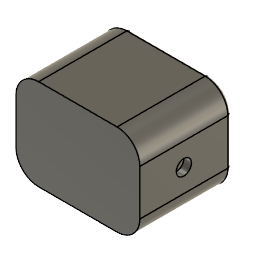
gimbal (Autodesk Fusion 360 archive; units mm, degrees)
design "camera"
Autodesk Fusion 360 part; units mm, degrees
sketch "Sketch1" plane through (0, 0, 0) normal (0, 0, 1) x (1, 0, 0)
  line L0 (20.4, -15) -> (-20.4, -15)
  line L1 (-20.4, -15) -> (-20.4, 15)
  line L2 (-20.4, 15) -> (20.4, 15)
  line L3 (20.4, 15) -> (20.4, -15)
  line L4 (20.4, -15) -> (-20.4, 15) construction
  line L5 (-20.4, -15) -> (20.4, 15) construction
  dimension "d1" = 30
  dimension "d2" = 40.8
  constraint horizontal L0
  constraint perpendicular L0 L1
  constraint parallel L0 L2
  constraint parallel L1 L3
  constraint coincident L4 origin
  constraint coincident L5 origin
  measures "d1" distance of L0.end L1.end
  measures "d2" distance of L1.end L2.end
extrude "Extrude1" add sketch "Sketch1" along normal blind 30 makes body 1
fillet "Fillet4" radius 7.5 4 edges at (20.4, 0, 30) (-20.4, 0, 30) (20.4, 0, 0) (-20.4, 0, 0) on bodies 1
hole "Hole1" at (0, 15, 15) direction (0, -1, 0) diameter 20 depth 15 tip angle 118 bodies 1
ref_plane "WorkPlane1" through (0, 20, 0) normal (0, 1, 0) x (0, 0, 1)
sketch "Sketch4" plane through (0, 15, 0) normal (0, 1, 0) x (-1, 0, 0)
  circle A0 centre (0, 15) radius 10
  arc A1 (12.9, 0) -> (20.4, 7.5) centre (12.9, 7.5) ccw
  line L0 (20.4, 7.5) -> (20.4, 22.5)
  arc A2 (20.4, 22.5) -> (12.9, 30) centre (12.9, 22.5) ccw
  line L1 (12.9, 30) -> (-12.9, 30)
  arc A3 (-12.9, 30) -> (-20.4, 22.5) centre (-12.9, 22.5) ccw
  line L2 (-20.4, 22.5) -> (-20.4, 7.5)
  arc A4 (-20.4, 7.5) -> (-12.9, 0) centre (-12.9, 7.5) ccw
  line L3 (-12.9, 0) -> (12.9, 0)
  circle A5 centre (0, 15) radius 10
  constraint concentric A0 A5
extrude "Extrude4" add sketch "Sketch4" along normal blind 1 separate body contours A0 A5 makes body 2
ref_plane "WorkPlane3" through (0, 16, 15) normal (0, 1, 0) x (-1, 0, 0)
sketch "Sketch5" plane through (0, 16, 0) normal (0, 1, 0) x (1, 0, 0)
  circle A0 centre (0, -15) radius 8.2462
extrude "Extrude5" add sketch "Sketch5" along normal blind 2 bodies 2
fillet "Fillet5" radius 0.9 1 edges at (-7.6882, 18, 17.982) on bodies 2
fillet "Fillet6" radius 0.4 1 edges at (9.3233, 16, 11.3838) on bodies 2
fillet "Fillet7" radius 1 1 faces at (-16.924, 15, 14.7509) on bodies 1
ref_plane "WorkPlane4" through (0, 15, 15) normal (0, 1, 0) x (-1, 0, 0)
sketch "Sketch6" plane through (0, 15, 0) normal (0, 1, 0) x (1, 0, 0)
  circle A0 centre (-13, -25) radius 2
  dimension "d42" = 4
  measures "d42" diameter of A0
extrude "Extrude6" cut sketch "Sketch6" against normal blind 0.5 bodies 1
hole "Hole2" at (20.4, -0.5, 15) direction (-1, 0, 0) diameter 5 depth 2.5 tip angle 180 bodies 1
hole "Hole3" at (-20.4, -0.5, 15) direction (1, 0, 0) diameter 5 depth 2.5 tip angle 180 bodies 1

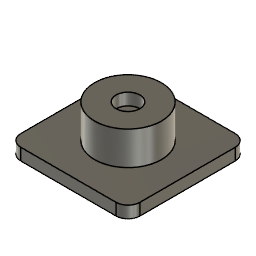
design "gimble stand"
Autodesk Fusion 360 part; units mm, degrees
sketch "Sketch1" plane through (0, 0, 0) normal (0, 0, 1) x (1, 0, 0)
  line L0 (25, -25) -> (-25, -25)
  line L1 (-25, -25) -> (-25, 25)
  line L2 (-25, 25) -> (25, 25)
  line L3 (25, 25) -> (25, -25)
  line L4 (25, -25) -> (-25, 25) construction
  line L5 (-25, -25) -> (25, 25) construction
  dimension "d1" = 50
  dimension "d2" = 50
  constraint horizontal L0
  constraint perpendicular L0 L1
  constraint parallel L0 L2
  constraint parallel L1 L3
  constraint coincident L4 origin
  constraint coincident L5 origin
  measures "d1" distance of L1.end L2.end
  measures "d2" distance of L0.end L1.end
extrude "Extrude1" add sketch "Sketch1" along normal blind 5
ref_plane "WorkPlane1" through (0, 0, 5) normal (0, 0, 1) x (1, 0, 0)
sketch "Sketch2" plane through (0, 0, 5) normal (0, 0, 1) x (1, 0, 0)
  circle A0 centre (0, 0) radius 14
  dimension "d6" = 28
  constraint coincident A0.centre origin
  measures "d6" diameter of A0
extrude "Extrude2" add sketch "Sketch2" along normal blind 14
ref_plane "WorkPlane2" through (0, 0, 19) normal (0, 0, 1) x (1, 0, 0)
sketch "Sketch3" plane through (0, 0, 19) normal (0, 0, 1) x (1, 0, 0)
  circle A0 centre (0, 0) radius 5
  dimension "d10" = 10
  constraint coincident A0.centre origin
  measures "d10" diameter of A0
extrude "Extrude3" cut sketch "Sketch3" against normal blind 5
fillet "Fillet1" radius 5 4 edges at (25, -25, 2.5) (-25, -25, 2.5) (25, 25, 2.5) (-25, 25, 2.5)

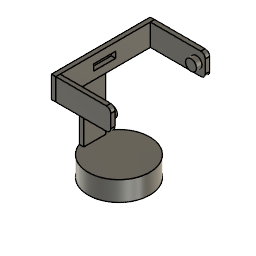
design "holder"
Autodesk Fusion 360 part; units mm, degrees
sketch "Sketch1" plane through (0, 0, 0) normal (0, 0, 1) x (1, 0, 0)
  circle A0 centre (0, 0) radius 14
  dimension "d1" = 28
  constraint coincident A0.centre origin
  measures "d1" diameter of A0
extrude "Extrude1" add sketch "Sketch1" along normal blind 14 makes body 1
ref_plane "WorkPlane1" through (0, -11, 0) normal (0, 1, 0) x (0, 0, 1)
ref_plane "WorkPlane2" through (0, 0, 14) normal (0, 0, 1) x (1, 0, 0)
sketch "Sketch2" plane through (0, 0, 14) normal (0, 0, 1) x (1, 0, 0)
  line L0 (-11, -5) -> (-13, -5)
  line L1 (-13, -5) -> (-13, 5)
  line L2 (-13, 5) -> (-11, 5)
  line L3 (-11, 5) -> (-11, -5)
  line L4 (-11, -5) -> (-13, 5) construction
  line L5 (-13, -5) -> (-11, 5) construction
  point P0 (-12, 0)
  constraint horizontal L0
  constraint perpendicular L0 L1
  constraint parallel L0 L2
  constraint parallel L1 L3
  constraint coincident L4 P0
  constraint coincident L5 P0
extrude "Extrude2" add sketch "Sketch2" along normal blind 35 bodies 1
ref_plane "WorkPlane5" through (-11, 0, 0) normal (1, 0, 0) x (0, 1, 0)
sketch "Sketch3" plane through (-11, 0, 0) normal (1, 0, 0) x (0, 1, 0)
  line L0 (5, 46.1306) -> (-5, 46.1306)
  line L1 (-5, 46.1306) -> (-5, 48.9328)
  line L2 (-5, 48.9328) -> (5, 48.9328)
  line L3 (5, 48.9328) -> (5, 46.1306)
  line L4 (5, 46.1306) -> (-5, 48.9328) construction
  line L5 (-5, 46.1306) -> (5, 48.9328) construction
  point P0 (0, 47.5317)
  constraint horizontal L0
  constraint perpendicular L0 L1
  constraint parallel L0 L2
  constraint parallel L1 L3
  constraint coincident L4 P0
  constraint coincident L5 P0
extrude "Extrude3" add sketch "Sketch3" along normal blind 2.5 bodies 1
fillet "Fillet1" radius 2.5 1 edges at (-13, 0, 49) on bodies 1
sketch "Sketch4" plane through (-8.5, 0, 0) normal (1, 0, 0) x (0, 1, 0)
  line L0 (5, 48.9328) -> (-5, 48.9328)
  line L1 (-5, 48.9328) -> (-5, 46.1306)
  line L2 (-5, 46.1306) -> (5, 46.1306)
  line L3 (5, 46.1306) -> (5, 48.9328)
  line L4 (22.7362, 52.5415) -> (-22.2638, 52.5415)
  line L5 (-22.2638, 52.5415) -> (-22.2638, 42.5415)
  line L6 (-22.2638, 42.5415) -> (22.7362, 42.5415)
  line L7 (22.7362, 42.5415) -> (22.7362, 52.5415)
  line L8 (22.7362, 52.5415) -> (-22.2638, 42.5415) construction
  line L9 (-22.2638, 52.5415) -> (22.7362, 42.5415) construction
  point P0 (0.2362, 47.5415)
  dimension "d15" = 10
  dimension "d16" = 45
  constraint horizontal L4
  constraint perpendicular L4 L5
  constraint parallel L4 L6
  constraint parallel L5 L7
  constraint coincident L8 P0
  constraint coincident L9 P0
  measures "d15" distance of L4.end L5.end
  measures "d16" distance of L5.end L6.end
extrude "Extrude4" add sketch "Sketch4" along normal blind 2 separate body makes body 2
sketch "Sketch6" plane through (0, 0, 0) normal (1, 0, 0) x (0, 1, 0)
ref_plane "WorkPlane6" through (-6.5, 0.2362, 47.5415) normal (1, 0, 0) x (0, 0, -1)
sketch "Sketch7" plane through (-6.5, 0, 0) normal (1, 0, 0) x (0, 1, 0)
  line L0 (22.7658, 42.5492) -> (20.7658, 42.5492)
  line L1 (20.7658, 42.5492) -> (20.7658, 52.5492)
  line L2 (20.7658, 52.5492) -> (22.7658, 52.5492)
  line L3 (22.7658, 52.5492) -> (22.7658, 42.5492)
  line L4 (22.7658, 42.5492) -> (20.7658, 52.5492) construction
  line L5 (20.7658, 42.5492) -> (22.7658, 52.5492) construction
  line L6 (-20.2334, 42.5492) -> (-22.2334, 42.5492)
  line L7 (-22.2334, 42.5492) -> (-22.2334, 52.5492)
  line L8 (-22.2334, 52.5492) -> (-20.2334, 52.5492)
  line L9 (-20.2334, 52.5492) -> (-20.2334, 42.5492)
  line L10 (-20.2334, 42.5492) -> (-22.2334, 52.5492) construction
  line L11 (-22.2334, 42.5492) -> (-20.2334, 52.5492) construction
  point P0 (21.7658, 47.5492)
  point P1 (-21.2334, 47.5492)
  dimension "d21" = 2
  dimension "d22" = 10
  dimension "d23" = 2
  dimension "d24" = 10
  constraint horizontal L0
  constraint perpendicular L0 L1
  constraint parallel L0 L2
  constraint parallel L1 L3
  constraint coincident L4 P0
  constraint coincident L5 P0
  constraint horizontal L6
  constraint perpendicular L6 L7
  constraint parallel L6 L8
  constraint parallel L7 L9
  constraint coincident L10 P1
  constraint coincident L11 P1
  measures "d21" distance of L1.end L2.end
  measures "d22" distance of L0.start L2.end
  measures "d23" distance of L7.end L8.end
  measures "d24" distance of L6.end L7.end
extrude "Extrude5" add sketch "Sketch7" along normal blind 25 bodies 2
fillet "Fillet2" radius 2 2 edges at (18.5, -21.2334, 42.5492) (18.5, -21.2334, 52.5492) on bodies 2
fillet "Fillet3" radius 2 2 edges at (18.5, 21.7658, 52.5492) (18.5, 21.7658, 42.5492) on bodies 2
ref_plane "WorkPlane7" through (6, 20.7658, 47.5492) normal (0, -1, 0) x (0, 0, -1)
sketch "Sketch8" plane through (0, 20.7658, 0) normal (0, -1, 0) x (-1, 0, 0)
  circle A0 centre (-14.6062, -47.2996) radius 2.5
  circle A1 through (-12.0757, -47.2508, 40.9991) (-15.8257, -45.0857, 40.9991) (-15.8257, -49.4158, 40.9991)
  dimension "d32" = 5
  dimension "d33" = 5
  measures "d32" diameter of A0
extrude "Extrude6" add sketch "Sketch8" against normal blind 2.5 contours A1 in plane through (0, -20.2333, 0) normal (0, -1, 0) bodies 2
ref_plane "WorkPlane8" through (6, 20.7658, 47.5492) normal (0, -1, 0) x (0, 0, -1)
sketch "Sketch9" plane through (0, 20.7658, 0) normal (0, -1, 0) x (-1, 0, 0)
  circle A0 centre (-14.5125, -47.3627) radius 2.5
  dimension "d37" = 5
  measures "d37" diameter of A0
extrude "Extrude7" add sketch "Sketch9" along normal blind 2.5 bodies 2
sketch "Sketch10" plane through (0, 0, 0) normal (0, 0, -1) x (1, 0, 0)
  circle A0 centre (0, 0) radius 14
  circle A1 centre (0, 0) radius 5
  dimension "d40" = 10
  constraint concentric A0 A1
  measures "d40" diameter of A1
extrude "Extrude8" cut sketch "Sketch10" against normal blind 5 bodies 1
